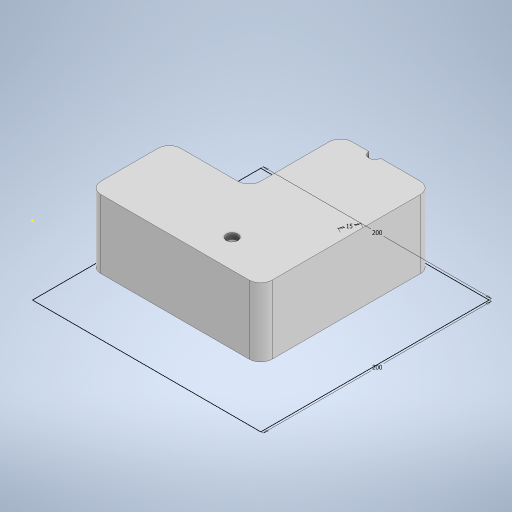
# Autodesk Inventor part: Area øh1
Saved by Autodesk Inventor 2024 (Build 280153000, 153)
## iProperties
Created: 2024-03-01
Part Number: Area øh1
Material: Generic
Document SubType Name: Modeling
Designer: laura
Density: 1 g/cm^3
Appearance: Default
Author: laura
Autodesk Inventor part; units mm, degrees
ref_plane "YZ Plane" through (0, 0, 0) normal (1, 0, 0) x (0, 1, 0)
ref_plane "XZ Plane" through (0, 0, 0) normal (0, 1, 0) x (-1, 0, 0)
ref_plane "XY Plane" through (0, 0, 0) normal (0, 0, 1) x (1, 0, 0)
sketch "Sketch1" plane through (0, 0, 0) normal (0, 1, 0) x (-1, 0, 0)
  line L0 (0, 0) -> (-200, 0)
  line L1 (-200, 0) -> (-200, -200)
  line L2 (-200, -200) -> (0, -200)
  line L3 (0, -200) -> (0, 0)
  line L4 (-89.8726, -200) -> (-110.1274, -200)
  line L5 (-114.7696, -186.0054) -> (-100, -186.0054)
  line L6 (-110.1274, -200) -> (-115.8572, -187.7125)
  arc A0 (-114.7696, -186.0054) -> (-115.8572, -187.7125) centre (-114.7696, -187.2054) ccw
  line L7 (-100, -186.0054) -> (-85.2304, -186.0054)
  line L8 (-90, -199.8) -> (-90, -186.3697) construction
  arc A1 (-84.1428, -187.7125) -> (-85.2304, -186.0054) centre (-85.2304, -187.2054) ccw
  line L9 (-84.1428, -187.7125) -> (-89.8726, -200)
  line L10 (-0.2, -90) -> (13.2303, -90) construction
  arc A2 (12.0565, -115.4946) -> (13.1946, -114.7696) centre (12.3946, -114.7696) ccw
  line L11 (0, -109.8726) -> (12.0565, -115.4946)
  line L12 (0, -90.1274) -> (0, -109.8726)
  line L13 (13.1946, -114.7696) -> (13.1946, -100)
  line L14 (12.0565, -84.5054) -> (0, -90.1274)
  line L15 (13.1946, -100) -> (13.1946, -85.2304)
  arc A3 (13.1946, -85.2304) -> (12.0565, -84.5054) centre (12.3946, -85.2304) ccw
  point P0 (-100, -200)
  point P1 (-100, -200)
  point P2 (-100, -200)
  point P3 (-83.6607, -186.2054)
  point P4 (-100, -200)
  point P5 (0, -100)
  point P6 (0, -100)
  point P7 (0, -100)
  point P8 (0, -100)
  point P9 (0, -100)
  point P10 (0, -100)
  dimension "d0" = 200
  dimension "d1" = 200
  dimension "d2" = 15
  constraints: 32 end point, 8 point on circle, 4 centre point, 2 midpoint, 2 parallel, 1 horizontal, 1 perpendicular
  measures "d0" distance of L2.end L1.end
  measures "d1" distance of L1.end L0.end
  measures "d2" distance of L8.start point (-83.661, -186.205)
extrude "Extrusion1" add sketch "Sketch1" along normal blind 60 contours L3 L2 L9 A1 L7 L5 A0 L6 L1 L0 | L6 A0 L5 L7 A1 L9 L2
extrude "Extrusion3" cut sketch "Sketch1" along normal blind 5.2 contours L6 A0 L5 L7 A1 L9 L2
sketch "Sketch2" plane through (0, 60, 0) normal (0, 1, 0) x (1, 0, 0)
  point P0 (0, 0)
sketch "Sketch3" plane through (0, 60, 0) normal (0, 1, 0) x (1, 0, 0)
  line L0 (0, 0) -> (200, 0) projected
  circle A0 centre (100, 75) radius 5.1
  line L1 (200, 200) -> (0, 200) projected
  circle A1 centre (100, 200) radius 5.1
  dimension "d10" = 10.2
  dimension "d11" = 10.2
  constraints: 2 centre point, 1 midpoint
  measures "d10" diameter of A0
  measures "d11" diameter of A1
extrude "Extrusion4" cut sketch "Sketch3" against normal blind 5.2
extrude "Extrusion5" add sketch "Sketch1" along normal blind 4.8 contours L14 A3 L15 L13 A2 L11 L3
sketch "Sketch4" plane through (0, 60, 0) normal (0, 1, 0) x (1, 0, 0)
  line L0 (0, 200) -> (0, 0) projected
  line L1 (200, 0) -> (200, 200) projected
  line L2 (0, 0) -> (200, 0)
  line L3 (200, 0) -> (200, 50)
  line L4 (200, 50) -> (0, 50)
  line L5 (0, 50) -> (0, 0)
  line L6 (200, 200) -> (110.1274, 200) projected
  line L7 (200, 0) -> (130, 0)
  line L8 (130, 0) -> (130, 200)
  line L9 (130, 200) -> (200, 200)
  line L10 (200, 200) -> (200, 0)
  point P0 (130, 50)
  dimension "d16" = 50
  dimension "d17" = 70
  constraints: 16 end point, 4 parallel, 2 horizontal, 2 perpendicular, 2 point on line
  measures "d16" distance of L3.end L2.end
  measures "d17" distance of L8.end L9.end
extrude "Extrusion6" cut sketch "Sketch4" against normal blind 60
sketch "Sketch5" plane through (0, 0, 0) normal (0, -1, 0) x (1, 0, 0)
  line L0 (89.8726, -200) -> (0, -200) projected
  line L1 (0, -200) -> (70, -200)
  line L2 (70, -200) -> (70, -120)
  line L3 (70, -120) -> (0, -120)
  line L4 (0, -120) -> (0, -200)
  point P0 (0, 0)
  dimension "d20" = 70
  dimension "d21" = 80
  constraints: 8 end point, 2 parallel, 1 horizontal, 1 perpendicular
  measures "d20" distance of L3.end L2.end
  measures "d21" distance of L2.end L1.end
extrude "Extrusion7" cut sketch "Sketch5" against normal blind 60
sketch "Sketch6" plane through (130, 60, -50) normal (1, 0, 0) x (0, 0, -1)
  line L0 (0, 0) -> (0, -60) projected
  line L1 (150, -60) -> (0, -60) projected
  line L2 (0, 0) -> (150, 0)
  line L3 (150, 0) -> (150, -60)
  line L4 (150, -60) -> (0, -60)
  line L5 (0, -60) -> (0, 0)
  point P0 (-50, -60)
  constraints: 8 end point, 2 parallel, 1 horizontal, 1 perpendicular
extrude "Extrusion8" add sketch "Sketch6" along normal blind 20
fillet "Fillet2" radius 10 6 edges at (150, 30, -200) (70, 30, -200) (0, 30, -120) (150, 30, -50) (70, 30, -120) (0, 30, -50)
body "Solid1"
